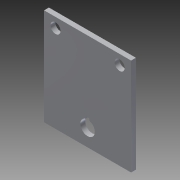
# Autodesk Inventor part: arm mout
Saved by Autodesk Inventor 2013 (Build 170138000, 138)
## iProperties
Created: 2013-01-24
Part Number: arm mout
Material: Aluminum 6061
Document SubType Name: Sheet Metal
Designer: Arpan
Density: 2.71 g/cm^3
Sheet Metal Rule: Default
Mass: 29.9392 g
Surface Area: 79.5108 cm^2
Volume: 11.0477 cm^3
Author: Arpan
Autodesk Inventor part; units mm, degrees
ref_plane "YZ Plane" through (0, 0, 0) normal (1, 0, 0) x (0, 1, 0)
ref_plane "XZ Plane" through (0, 0, 0) normal (0, 1, 0) x (-1, 0, 0)
ref_plane "XY Plane" through (0, 0, 0) normal (0, 0, 1) x (1, 0, 0)
sketch "Sketch1" plane through (0, 0, 0) normal (0, 0, 1) x (1, 0, 0)
  line L0 (-56.9976, 63.5) -> (0, 63.5)
  line L1 (0, 63.5) -> (-7.493, 63.5)
  line L2 (-7.493, 63.5) -> (-7.493, 57.15)
  line L3 (-56.9976, 63.5) -> (-49.5046, 63.5)
  line L4 (-49.5046, 63.5) -> (-49.5046, 57.15)
  circle A0 centre (-49.5046, 57.15) radius 3.302
  circle A1 centre (-7.493, 57.15) radius 3.302
  line L5 (-56.9976, 63.5) -> (-56.9976, 0)
  line L6 (-56.9976, 0) -> (0, 0)
  line L7 (0, 0) -> (0, 63.5)
  line L8 (-28.4988, 0) -> (-28.4988, 11.1125)
  circle A2 centre (-28.4988, 11.1125) radius 4.7625
  dimension "d3" = 7.493
  dimension "d4" = 6.35
  dimension "d5" = 7.493
  dimension "d6" = 6.604
  dimension "d7" = 6.604
  dimension "d19" = 6.35
  dimension "d60" = 63.5
  dimension "d61" = 11.1125
  dimension "d62" = 9.525
  constraints: 18 end point, 3 centre point, 3 coincident, 3 perpendicular, 2 point on line, 1 midpoint, 1 parallel
  measures "d3" distance of L0.end L1.end
  measures "d4" distance of L1.end L2.end
  measures "d5" distance of L0.start L3.end
  measures "d6" diameter of A0
  measures "d7" diameter of A1
  measures "d19" distance of L3.end L4.end
  measures "d60" distance of L0.start L5.end
  measures "d61" distance of L8.start L8.end
  measures "d62" diameter of A2
extrude "Plate6" add sketch "Sketch1" along normal blind 3.175
sketch "Sketch6" plane through (0, 0, 0) normal (0, 0, -1) x (-1, 0, 0)
  circle A0 centre (28.4988, 11.1125) radius 4.7625 projected
  line L0 (0, 63.5) -> (56.9976, 63.5) projected
  line L1 (28.4988, 15.875) -> (29.6894, 15.875)
  line L2 (28.4988, 15.875) -> (27.305, 15.875)
  line L3 (27.305, 15.875) -> (27.305, 17.0656)
  line L4 (27.305, 17.0656) -> (29.6894, 17.0656)
  line L5 (29.6894, 17.0656) -> (29.6894, 15.875)
  line L6 (27.305, 15.875) -> (27.305, 15.7229)
  line L7 (29.6894, 15.875) -> (29.6894, 15.7238)
  dimension "d64" = 1.1906
  dimension "d65" = 1.1938
  dimension "d66" = 1.1906
  constraints: 14 end point, 5 parallel, 3 point on circle, 2 tangent, 1 collinear, 1 perpendicular
  measures "d64" distance of L1.start L1.end
  measures "d65" distance of L1.start L2.end
  measures "d66" distance of L2.end L3.end
extrude "Cut1" cut sketch "Sketch6" against normal blind 3.175 contours A0 L1 L7 | L6 L2 A0 | L2 L3 L4 L5 L1
equation "\"d67\" = Thickness"
equation "\"BendRadius\" = Thickness"
equation "\"BendReliefWidth\" = Thickness"
equation "\"BendReliefDepth\" = 0.5 * Thickness"
equation "\"CornerReliefSize\" = 4 * Thickness"
equation "\"MinimumRemnant\" = 2 * Thickness"
equation "\"TransitionRadius\" = BendRadius"
equation "\"JacobiRadiusSize\" = BendRadius"
equation "\"GapSize\" = Thickness"
equation "\"d8\" = BendRadius"
equation "\"d56\" = BendRadius"
equation "\"d63\" = BendRadius"
equation "\"Thickness\" = 3.175"
body "Solid3"
